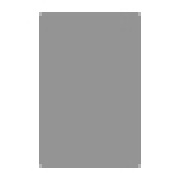
# Autodesk Inventor part: Platte Scharfe Ecken (mm) 150 x 30 x 8
Saved by Autodesk Inventor 2025 (Build 290162010, 162A)
## iProperties
IsCustomPart: 1
Created: 2024-01-20
Part Number: Platte Scharfe Ecken (mm) 150 x 30 x 8
Material: Stahl, weich
Document SubType Name: Modeling
Designer: Admin
Language: de-DE
Size Designation: 150 x 30 x 8
Categories: <MemberInstance><Categories><Category DisplayName="Sonstige Bauteile" InternalName="5aa15e00-363f-49f2-933f-16f664388e3f" Mnemonic="OTHER"><Category DisplayName="Platten" InternalName="68c93ff6-4e8d-4eb7-8f6b-7193118faa00" Mnemonic="ENDCPS"><CategoryParameter DisplayName="Dicke" InternalName="9be01ee9-2b90-4dd5-b218-41fb7aa436e5" Mnemonic="THICKNESS"/><Category DisplayName="Rechteckig" InternalName="7fbb2c3d-3161-40ec-a69e-d88557b9a03d" Mnemonic="RECTENDCPS"><CategoryParameter DisplayName="Fase" InternalName="27fa188d-6fef-4c28-a142-8b3beccff299" Mnemonic="chamfer"/><CategoryParameter DisplayName="Höhe" InternalName="3f3587fd-b77f-4a19-8908-2b2cf8a6220a" Mnemonic="HEIGHT"/><CategoryParameter DisplayName="Rundung" InternalName="c4c2cad8-1734-4792-a2b6-b222e9e5dbda" Mnemonic="fillet"/><CategoryParameter DisplayName="Breite" InternalName="c685a2dc-1f68-4190-a4f4-cc4dc8ffa73f" Mnemonic="WIDTH"/></Category></Category></Category><Category DisplayName="Datentyp" InternalName="23b78d0f-2648-40c6-8793-ca6db495c9e8" Mnemonic="DATATYPE"><CategoryParameter DisplayName="Anzeigename" InternalName="05415f3d-3907-474b-a020-eb9d644f4cf3" Mnemonic="DISPLAYNAME"/><CategoryParameter DisplayName="Norm" InternalName="0c0a119c-1e12-4c84-803f-101930972f5e" Mnemonic="STANDARD"/><CategoryParameter DisplayName="Beschreibung" InternalName="13903e3d-64b1-4950-80da-f627842ea37f" Mnemonic="DESCRIPTION"/><CategoryParameter DisplayName="Bezeichnung" InternalName="2675968c-4ce5-49e0-a4f5-552d29089031" Mnemonic="DESIGNATION"/><CategoryParameter DisplayName="Standardzeile" InternalName="2af9ec52-faaa-4026-b378-f9fa4afca842" Mnemonic="DEFAULTROW"/><CategoryParameter DisplayName="Ordnername" InternalName="3f06958e-8713-4116-9be7-ed6184ecc97b" Mnemonic="FOLDERNAME"/><CategoryParameter DisplayName="Revisionsanleitung" InternalName="45a75005-10b1-4dfc-8d6d-dfe629f0b93c" Mnemonic="REVISIONGUID"/><CategoryParameter DisplayName="Dateiname" InternalName="8b46a4cc-9585-4fed-90c3-899f57e09a73" Mnemonic="FILENAME"/><CategoryParameter DisplayName="Normungsorganisation" InternalName="8f5914e1-4693-403f-8ab5-d37768198c9d" Mnemonic="STDSORG"/><CategoryParameter DisplayName="Gruppenversion" InternalName="914462f6-6e19-4b14-ba84-155b9680b1d0" Mnemonic="FAMILYREVISION"/><CategoryParameter DisplayName="Normrevision" InternalName="91d5a463-65c2-4fde-b823-3b7fea5e8e17" Mnemonic="STANDARDREVISION"/><CategoryParameter DisplayName="Variantenrevision" InternalName="a65d44b9-392f-4f4f-857b-e4b3d54996fe" Mnemonic="MEMBERREVISION"/><CategoryParameter DisplayName="ClipFormat" InternalName="bc51e27b-3422-4e78-93ef-cec197ddf230" Mnemonic="CLIPFORMAT"/><CategoryParameter DisplayName="Hersteller" InternalName="cd6c7a72-a28a-4e50-99a9-2c7f4e13e5ad" Mnemonic="MANUFACTURER"/><CategoryParameter DisplayName="InternerName" InternalName="cf1d0246-76d9-4b4a-8305-fa0409afb5c1" Mnemonic="INTERNALNAME"/><CategoryParameter DisplayName="IstMetrisch" InternalName="e2385c5b-1ea4-4823-96a8-8de651266ec3" Mnemonic="ISMETRIC"/><Category DisplayName="Bauteil" InternalName="c0e0b642-3bcb-4cc8-9e80-f96d35c4afa4" Mnemonic="PART"><CategoryParameter DisplayName="Bauteilnummer" InternalName="016b6077-bfbe-49bd-92c9-d8d59c39c941" Mnemonic="PARTNUMBER"/><CategoryParameter DisplayName="Bestandsnummer" InternalName="4dba7c1c-e26c-444e-836c-b08b433409a8" Mnemonic="STOCKNUMBER"/><CategoryParameter DisplayName="Materialschlüssel" InternalName="5c9a8adb-dd2b-4535-b97f-0a94a95fe41f" Mnemonic="MATERIALKEY"/><CategoryParameter DisplayName="Material" InternalName="818a152a-d3c3-49ca-80ee-df7d91421b8e" Mnemonic="MATERIAL"/></Category></Category></Categories><FamilyTemplate Id="Rectangular_mm"><FamilyTemplateParameters><FamilyTemplateParameter ObjectType="kUserParameterObject" ValueType="xs:double" Id="14" ObjectReferenceKey="height"/><FamilyTemplateParameter ObjectType="kUserParameterObject" ValueType="xs:double" Id="15" ObjectReferenceKey="thickness"/><FamilyTemplateParameter ObjectType="kUserParameterObject" ValueType="xs:double" Id="16" ObjectReferenceKey="width"/><FamilyTemplateParameter ObjectType="kPartComponentDefinitionObject" ValueType="xs:string" Id="27" SubObjectId="Material"/><FamilyTemplateParameter ObjectType="kPropertyObject" ValueType="xs:string" Id="31" ObjectReferenceKey="{32853F0F-3444-11d1-9E93-0060B03C1CA6}" SubObjectId="5"/><FamilyTemplateParameter ObjectType="kPropertyObject" ValueType="xs:string" Id="32" ObjectReferenceKey="{32853F0F-3444-11d1-9E93-0060B03C1CA6}" SubObjectId="52"/></FamilyTemplateParameters></FamilyTemplate><CategoryParameterMap><ParamToTemplateMap><ParamToTemplate CategoryParameter="//CategoryParameter[@InternalName='cf1d0246-76d9-4b4a-8305-fa0409afb5c1']" ConstantValue="84115669-66ca-45e0-ba2c-7be7af1a5676"/><ParamToTemplate CategoryParameter="//CategoryParameter[@InternalName='45a75005-10b1-4dfc-8d6d-dfe629f0b93c']" ConstantValue="b27d57ab-e732-4bad-870e-63dd057e8d3f"/><ParamToTemplate CategoryParameter="//CategoryParameter[@InternalName='3f06958e-8713-4116-9be7-ed6184ecc97b']" ConstantValue="Sharp Corners (mm)"/><ParamToTemplate CategoryParameter="//CategoryParameter[@InternalName='8f5914e1-4693-403f-8ab5-d37768198c9d']" TemplateParameter="21"/><ParamToTemplate CategoryParameter="//CategoryParameter[@InternalName='0c0a119c-1e12-4c84-803f-101930972f5e']" TemplateParameter="22"/><ParamToTemplate CategoryParameter="//CategoryParameter[@InternalName='91d5a463-65c2-4fde-b823-3b7fea5e8e17']" TemplateParameter="23"/><ParamToTemplate CategoryParameter="//CategoryParameter[@InternalName='cd6c7a72-a28a-4e50-99a9-2c7f4e13e5ad']" TemplateParameter="24"/><ParamToTemplate CategoryParameter="//CategoryParameter[@InternalName='13903e3d-64b1-4950-80da-f627842ea37f']" TemplateParameter="26"/><ParamToTemplate CategoryParameter="//CategoryParameter[@InternalName='05415f3d-3907-474b-a020-eb9d644f4cf3']" ConstantValue="Sharp Corners (mm)"/><ParamToTemplate CategoryParameter="//CategoryParameter[@InternalName='914462f6-6e19-4b14-ba84-155b9680b1d0']" ConstantValue="11"/><ParamToTemplate CategoryParameter="//CategoryParameter[@InternalName='bc51e27b-3422-4e78-93ef-cec197ddf230']" ConstantValue="CF_INVENTOR.STDPARTS"/><ParamToTemplate CategoryParameter="//CategoryParameter[@InternalName='e2385c5b-1ea4-4823-96a8-8de651266ec3']" ConstantValue="true"/><ParamToTemplate CategoryParameter="//CategoryParameter[@InternalName='2af9ec52-faaa-4026-b378-f9fa4afca842']" ConstantValue="1"/><ParamToTemplate CategoryParameter="//CategoryParameter[@InternalName='8b46a4cc-9585-4fed-90c3-899f57e09a73']" ConstantValue="Platte Scharfe Ecken (mm) 150 x 30 x 8"/><ParamToTemplate CategoryParameter="//CategoryParameter[@InternalName='a65d44b9-392f-4f4f-857b-e4b3d54996fe']" ConstantValue="7DC41C41-53BF-4733-9A73-DC1655548DDD"/><ParamToTemplate CategoryParameter="//CategoryParameter[@InternalName='a65d44b9-392f-4f4f-857b-e4b3d54996fe']" ConstantValue="7DC41C41-53BF-4733-9A73-DC1655548DDD"/><ParamToTemplate CategoryParameter="//CategoryParameter[@InternalName='2675968c-4ce5-49e0-a4f5-552d29089031']" TemplateParameter="32"/><ParamToTemplate CategoryParameter="//CategoryParameter[@InternalName='818a152a-d3c3-49ca-80ee-df7d91421b8e']" TemplateParameter="27"/><ParamToTemplate CategoryParameter="//CategoryParameter[@InternalName='016b6077-bfbe-49bd-92c9-d8d59c39c941']" TemplateParameter="31"/><ParamToTemplate CategoryParameter="//CategoryParameter[@InternalName='3f3587fd-b77f-4a19-8908-2b2cf8a6220a']" TemplateParameter="14"/><ParamToTemplate CategoryParameter="//CategoryParameter[@InternalName='9be01ee9-2b90-4dd5-b218-41fb7aa436e5']" TemplateParameter="15"/><ParamToTemplate CategoryParameter="//CategoryParameter[@InternalName='c685a2dc-1f68-4190-a4f4-cc4dc8ffa73f']" TemplateParameter="16"/></ParamToTemplateMap></CategoryParameterMap></MemberInstance>
Density: 7.85 g/cm^3
Appearance: Halbpoliert
Author: Admin
Autodesk Inventor part; units mm, degrees
ref_plane "YZ Plane" through (0, 0, 0) normal (1, 0, 0) x (0, 1, 0)
ref_plane "XZ Plane" through (0, 0, 0) normal (0, 1, 0) x (-1, 0, 0)
ref_plane "XY Plane" through (0, 0, 0) normal (0, 0, 1) x (1, 0, 0)
sketch "Sketch1" plane through (0, 0, 0) normal (0, 0, 1) x (1, 0, 0)
  line L0 (0, 20.1746) -> (0, -21.4461) construction
  line L1 (-20.2028, 0) -> (20.1685, 0) construction
  line L2 (-100, 12) -> (100, 12)
  line L3 (100, 12) -> (100, -12)
  line L4 (100, -12) -> (-100, -12)
  line L5 (-100, -12) -> (-100, 12)
  point P0 (0, 0)
  dimension "d0" = 24
  dimension "d1" = 12
  dimension "d2" = 200
  dimension "d3" = 100
  constraints: 12 end point, 2 horizontal, 2 parallel, 2 point on line, 1 perpendicular, 1 vertical
  measures "d0" distance between parallel lines of L4 L2
  measures "d1" distance between parallel lines of L1 L2
  measures "d2" distance between parallel lines of L5 L3
  measures "d3" distance between parallel lines of L5 L0
extrude "Extrusion1" add sketch "Sketch1" along normal blind 8
fillet "Fillet1" [suppressed]
chamfer "Chamfer1" [suppressed]
sketch "Skizze2" plane through (0, 0, 8) normal (0, 0, 1) x (1, 0, 0)
  line L0 (-7.5, 0) -> (7.5, 0)
  point P0 (0, 0)
  point P1 (0, 0)
  dimension "d12" = 15
  constraints: 3 coincident, 2 end point, 1 horizontal, 1 midpoint
  measures "d12" distance of L0.start L0.end
sketch "Skizze3" plane through (0, 0, 8) normal (0, 0, 1) x (1, 0, 0)
  line L0 (-35, 0) -> (35, 0) construction
  point P0 (0, 0)
  point P1 (0, 0)
  dimension "d13" = 70
  constraints: 2 end point, 1 coincident, 1 horizontal, 1 midpoint
  measures "d13" distance of L0.end L0.start
hole "Bohrung1" at (-35, 0, 8) at (35, 0, 8) direction (0, 0, -1) diameter 5.3 end through all clearance for "Sechskantkopfschraube" size "M5" standard "ANSI Metrisches M Profil"
hole "Bohrung2" at (-7.5, 0, 8) at (7.5, 0, 8) direction (0, 0, -1) diameter 4.134 end through all start extended yes thread size "M5x0.8" class "6H" standard "ANSI Metric M Profile"
sketch "Skizze4" plane through (0, 0, 8) normal (0, 0, 1) x (1, 0, 0)
  circle A0 centre (-46, 0) radius 1.6 projected
  circle A1 centre (-23.5, 0) radius 1.6 projected
  circle A2 centre (46, 0) radius 1.6 projected
  circle A3 centre (23.5, 0) radius 1.6 projected
  point P0 (0, 0)
hole "Bohrung3" at (23.5, 0, 8) at (46, 0, 8) at (-23.5, 0, 8) at (-46, 0, 8) direction (0, 0, -1) diameter 2.459 end through all start extended yes thread size "M3x0.5" class "6H" standard "ANSI Metric M Profile"
sketch "Skizze5" plane through (0, 0, 8) normal (0, 0, 1) x (1, 0, 0)
  line L0 (-100, 6) -> (-50, 6)
  line L1 (-50, 6) -> (-50, -6)
  line L2 (-50, -6) -> (-100, -6)
  line L3 (-100, -6) -> (-100, 6)
  line L4 (-100, 12) -> (-100, -12) projected
  line L5 (-50, -6) -> (-50, -12)
  line L6 (-50, 6) -> (-50, 12)
  line L7 (100, 12) -> (-100, 12) projected
  line L8 (-50, 12) -> (-100, 12)
  line L9 (-100, -12) -> (100, -12) projected
  line L10 (-50, -12) -> (-100, -12)
  line L11 (0, 12) -> (0, -12)
  line L12 (100, 6) -> (50, 6)
  line L13 (50, 6) -> (50, -6)
  line L14 (50, -6) -> (100, -6)
  line L15 (100, -6) -> (100, 6)
  line L16 (100, 12) -> (100, -12)
  line L17 (50, -6) -> (50, -12)
  line L18 (50, 6) -> (50, 12)
  line L19 (50, 12) -> (100, 12)
  line L20 (50, -12) -> (100, -12)
  point P0 (0, 0)
  point P1 (-100, 0)
  point P2 (-100, 6)
  point P3 (100, 0)
  point P4 (50, -12)
  point P5 (50, 12)
  dimension "d35" = 50
  dimension "d36" = 12
  constraints: 36 end point, 7 symmetric about line, 4 midpoint, 2 collinear, 2 parallel, 1 horizontal, 1 perpendicular, 1 vertical
  measures "d35" distance of L1.end L2.end
  measures "d36" distance of L0.end L1.end
extrude "Extrusion2" cut sketch "Skizze5" against normal through all contours L4 L7 L6 L0 | L2 L5 L9 L4 | L7 L16 L12 L18 | L17 L14 L16 L9
fillet "Rundung2" radius 3 4 edges at (-75, -6, 8) (-75, 6, 8) (75, 6, 8) (75, -6, 8)
equation "\"d0\" = height"
equation "\"d1\" = 0.5 * height"
equation "\"d2\" = width"
equation "\"d3\" = 0.5 * width"
equation "\"d4\" = thickness"
equation "\"fillet\" = 0"
equation "\"chamfer\" = 0"
equation "\"thickness\" = 8"
equation "\"width\" = 200"
equation "\"height\" = 24"
body "Solid1"
